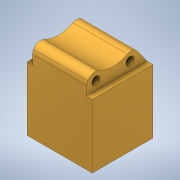
# Autodesk Inventor part: Kauri modular session 5 mount
Saved by Autodesk Inventor 2020 (Build 240168000, 168)
## iProperties
Created: 2022-05-05
Part Number: Kauri modular session 5 mount
Material: Brass, Soft Yellow
Document SubType Name: Modeling
Designer: Steven
Density: 8.47 g/cm^3
Appearance: Brass - Satin
Mass: 18.7081 g
Surface Area: 16.7722 cm^2
Volume: 2.20875 cm^3
Author: Steven
Autodesk Inventor part; units mm, degrees
ref_plane "YZ Plane" through (0, 0, 0) normal (1, 0, 0) x (0, 1, 0)
ref_plane "XZ Plane" through (0, 0, 0) normal (0, 1, 0) x (-1, 0, 0)
ref_plane "XY Plane" through (0, 0, 0) normal (0, 0, 1) x (1, 0, 0)
sketch "Sketch1" plane through (0, 0, 0) normal (1, 0, 0) x (0, 1, 0)
  circle A0 centre (-9.7574, -19.7073) radius 1.55 construction
  circle A1 centre (0, 0) radius 1.55 construction
  circle A2 centre (-9.7574, -19.7073) radius 2.65
  circle A3 centre (0, 0) radius 2.65
  line L0 (-6.0684, -24.2876) -> (12.7398, 12.1607) construction
  arc A4 (-12.2239, -24.4871) -> (-4.9776, -22.1738) centre (-9.7574, -19.7073) ccw
  circle A5 centre (0, 0) radius 5.7448
  line L1 (-4.9776, -22.1738) -> (5.1052, -2.6344)
  arc A6 (-4.9776, -22.1738) -> (-12.2239, -24.4871) centre (-9.7574, -19.7073) ccw
  line L2 (-14.5372, -17.2408) -> (-5.1904, 2.4623)
  line L3 (0, 0) -> (0, -27.0135) construction
  line L4 (0, 0) -> (-9.7574, -19.7073) construction
  point P0 (-10.1101, -25.5779)
  dimension "d0" = 5.3
  dimension "d1" = 5.3
  dimension "d3" = 11.4897
  dimension "d4" = 5.3787
  dimension "d5" = 21.8076
  dimension "d6" = 21.9875
  constraints: 10 end point, 7 centre point, 7 point on circle, 4 coincident, 2 tangent, 1 point on line, 1 vertical
  measures "d0" diameter of A2
  measures "d1" diameter of A3
  measures "d3" diameter of A5
  measures "d4" radius of A6
  measures "d5" distance of L2.start L2.end
  measures "d6" distance of L1.start L1.end
extrude "Extrusion1" [suppressed]
sketch "Sketch4" plane through (0, 0, 0) normal (1, 0, 0) x (0, 1, 0)
  circle A0 centre (0, 0) radius 2.65 projected
  circle A1 centre (0, 0) radius 5.7448 projected
  line L0 (5.7448, 0) -> (5.7448, -21.991)
  line L1 (0, 0) -> (-9.7574, -19.7073) construction
  line L2 (5.7448, -21.991) -> (0, -21.991) construction
  circle A2 centre (0, -21.991) radius 5.7448
  circle A3 centre (0, -21.991) radius 2.65
  line L3 (-5.7448, -21.991) -> (-5.7448, 0)
  dimension "d22" = 21.991
  dimension "d23" = 21.9905
  dimension "d24" = 5.3
  constraints: 6 end point, 4 point on circle, 2 centre point, 2 coincident, 2 tangent, 1 horizontal, 1 vertical
  measures "d22" distance of L0.start L0.end
  measures "d23" distance of L1.start L1.end
  measures "d24" diameter of A3
extrude "Extrusion4" add sketch "Sketch4" along normal mid plane 35
sketch "Sketch6" plane through (0, 0, 0) normal (1, 0, 0) x (0, 1, 0)
  line L0 (5.7448, 0) -> (5.7448, -21.991) construction
  arc A0 (-5.7448, -21.991) -> (5.7448, -21.991) centre (0, -21.991) ccw construction
  line L1 (-5.7448, -21.991) -> (-5.7448, 0) construction
  arc A1 (5.7448, 0) -> (-5.7448, 0) centre (0, 0) ccw construction
  circle A2 centre (0, -21.991) radius 2.65 construction
  circle A3 centre (0, 0) radius 2.65 construction
  arc A4 (5.7448, 0) -> (-5.7448, 0) centre (0, 0) ccw construction
  line L2 (0, 0) -> (-5.7448, 0) construction
  line L3 (0, 5.7448) -> (-5.7448, 5.7448) construction
  line L4 (-5.7448, 5.7448) -> (-5.7448, -33.2552) construction
  line L5 (-5.7448, 5.7448) -> (-46.9448, 5.7448) construction
  line L6 (-5.7448, -33.2552) -> (-46.9448, -33.2552)
  line L7 (-46.9448, -33.2552) -> (-46.9448, 5.7448)
  line L8 (-46.9448, 5.7448) -> (-5.7448, 5.7448)
  line L9 (-5.7448, 5.7448) -> (-5.7448, -33.2552)
  dimension "d32" = 39
  dimension "d35" = 41.2
  constraints: 16 end point, 4 horizontal, 2 parallel, 1 perpendicular, 1 point on circle, 1 tangent, 1 vertical
  measures "d32" distance of L3.end L4.end
  measures "d35" distance of L3.end L5.end
extrude "Extrusion5" add sketch "Sketch6" along normal mid plane 42
sketch "Sketch7" plane through (17.5, 0, 0) normal (1, 0, 0) x (0, 0, -1)
  line L0 (21.991, 5.7448) -> (0, 5.7448) projected
  arc A0 (0, 5.7448) -> (0, -5.7448) centre (0, 0) ccw projected
  line L1 (0, -5.7448) -> (21.991, -5.7448) projected
  arc A1 (21.991, -5.7448) -> (21.991, 5.7448) centre (21.991, 0) ccw projected
  circle A2 centre (21.991, 0) radius 2.65 projected
  circle A3 centre (0, 0) radius 2.65 projected
  line L2 (-5.7448, -46.9448) -> (33.2552, -46.9448) projected
  line L3 (33.2552, -46.9448) -> (33.2552, -5.7448) projected
  line L4 (33.2552, -5.7448) -> (-5.7448, -5.7448) projected
  line L5 (-5.7448, -5.7448) -> (-5.7448, -46.9448) projected
  line L6 (33.2552, -5.7448) -> (26.6413, 3.3732)
  arc A4 (21.991, -5.7448) -> (21.991, 5.7448) centre (21.991, 0) ccw projected
  line L7 (-5.7448, -5.7448) -> (-5.7448, 0)
  arc A5 (0, 5.7448) -> (0, -5.7448) centre (0, 0) ccw projected
  point P0 (26.6413, 3.3732)
  point P1 (0, -5.7448)
  constraints: 4 end point, 3 point on circle, 1 tangent
extrude "Extrusion6" add sketch "Sketch7" against normal up to surface (35 mm away) contours A1 L1 A0 L0 | L6 L4 A1 | A0 L4 L7
sketch "Sketch8" plane through (17.5, 0, 0) normal (1, 0, 0) x (0, 0, -1)
  line L0 (21.991, 5.7448) -> (0, 5.7448) projected
  arc A0 (0, 5.7448) -> (-5.7448, 0) centre (0, 0) ccw projected
  line L1 (-5.7448, 0) -> (-5.7448, -5.7448) projected
  line L2 (33.2552, -5.7448) -> (-5.7448, -5.7448) projected
  line L3 (33.2552, -5.7448) -> (26.6413, 3.3732) projected
  arc A1 (26.6413, 3.3732) -> (21.991, 5.7448) centre (21.991, 0) ccw projected
  circle A2 centre (21.991, 0) radius 2.65 projected
  circle A3 centre (0, 0) radius 2.65 projected
  line L4 (0, 5.7448) -> (21.991, 5.7448) projected
  arc A4 (26.6413, 3.3732) -> (21.991, 5.7448) centre (21.991, 0) ccw projected
  arc A5 (0, 5.7448) -> (21.991, 5.7448) centre (10.9955, 22.4511) ccw
  dimension "d39" = 20
  constraints: 2 point on circle, 1 centre point
  measures "d39" radius of A5
extrude "Extrusion7" cut sketch "Sketch8" against normal up to next contours A5 L0
fillet "Fillet1" radius 5 2 edges at (0, 5.7448, -21.991) (0, 5.7448, 0)
body "Solid1"
